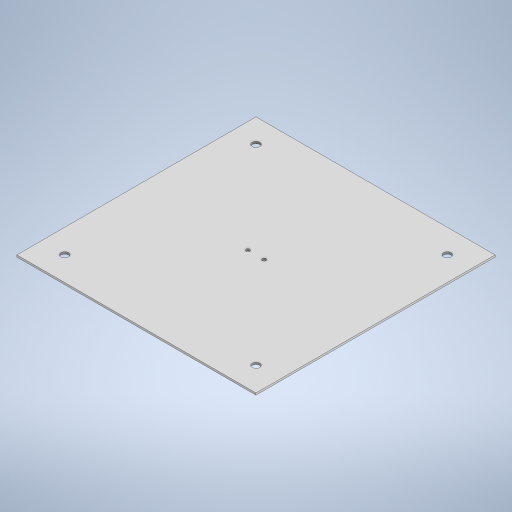
# Autodesk Inventor part: Пластина
Saved by Autodesk Inventor 2023 (Build 270158000, 158)
## iProperties
Created: 2022-05-06
Part Number: Пластина
Material: Типовые
Document SubType Name: Modeling
Designer: avkap
Density: 1 g/cm^3
Appearance: По умолчанию
Author: avkap
Autodesk Inventor part; units mm, degrees
ref_plane "YZ Plane" through (0, 0, 0) normal (1, 0, 0) x (0, 1, 0)
ref_plane "XZ Plane" through (0, 0, 0) normal (0, 1, 0) x (-1, 0, 0)
ref_plane "XY Plane" through (0, 0, 0) normal (0, 0, 1) x (1, 0, 0)
sketch "Эскиз1" plane through (0, 0, 0) normal (0, 1, 0) x (-1, 0, 0)
  line L0 (0, 0) -> (-250, 0)
  line L1 (-250, 0) -> (-250, -250)
  line L2 (-250, -250) -> (0, -250)
  line L3 (0, -250) -> (0, 0)
  line L4 (0, 0) -> (-25, 0)
  line L5 (-25, 0) -> (-25, -25)
  line L6 (-25, -25) -> (0, -25)
  line L7 (0, -25) -> (0, 0)
  line L8 (-250, -250) -> (-225, -250)
  line L9 (-225, -250) -> (-225, -225)
  line L10 (-225, -225) -> (-250, -225)
  line L11 (-250, -225) -> (-250, -250)
  line L12 (-225, -225) -> (-25, -225)
  line L13 (-25, -225) -> (-25, -25)
  line L14 (-25, -25) -> (-225, -25)
  line L15 (-225, -25) -> (-225, -225)
  circle A0 centre (-25, -25) radius 4
  circle A1 centre (-25, -225) radius 4
  circle A2 centre (-225, -25) radius 4
  circle A3 centre (-225, -225) radius 4
  line L16 (-250, -125) -> (0, -125)
  line L17 (-125, -125) -> (-116.5, -125)
  line L18 (-116.5, -125) -> (-133.5, -125)
  circle A4 centre (-116.5, -125) radius 2
  circle A5 centre (-133.5, -125) radius 2
  dimension "d0" = 250
  dimension "d1" = 250
  dimension "d2" = 25
  dimension "d3" = 25
  dimension "d4" = 25
  dimension "d5" = 25
  dimension "d6" = 8
  dimension "d7" = 8
  dimension "d8" = 8
  dimension "d9" = 8
  dimension "d10" = 8.5
  dimension "d11" = 17
  dimension "d12" = 4
  dimension "d13" = 4
  constraints: 38 end point, 8 parallel, 6 centre point, 6 coincident, 4 horizontal, 4 perpendicular, 3 midpoint, 2 point on line
  measures "d0" distance of L2.end L1.end
  measures "d1" distance of L1.end L0.end
  measures "d2" distance of L6.end L5.end
  measures "d3" distance of L5.end L4.end
  measures "d4" distance of L10.end L9.end
  measures "d5" distance of L9.end L8.end
  measures "d6" diameter of A0
  measures "d7" diameter of A1
  measures "d8" diameter of A2
  measures "d9" diameter of A3
  measures "d10" distance of L17.start L17.end
  measures "d11" distance of L17.end L18.end
  measures "d12" diameter of A4
  measures "d13" diameter of A5
extrude "Выдавливание1" add sketch "Эскиз1" along normal blind 2 contours L3 L6 A0 L5 L0 | L5 A0 L14 A2 L15 L16 L1 L0 | L3 L16 L13 A0 L6 | L3 L2 L9 A3 L12 A1 L13 L16 | L16 L15 A3 L10 L1 | A0 L13 L16 A4 A5 L15 A2 L14 | L13 A1 L12 A3 L15 L16 A5 A4 | L10 A3 L9 L2 L1
